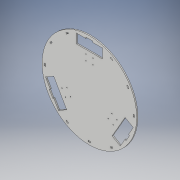
# Autodesk Inventor part: debanhxe
Saved by Autodesk Inventor 2019 (Build 230136000, 136)
## iProperties
Created: 2021-01-15
Part Number: debanhxe
Material: Generic
Document SubType Name: Modeling
Designer: Admin
Density: 1 g/cm^3
Appearance: Default
Author: Admin
Autodesk Inventor part; units mm, degrees
ref_plane "YZ Plane" through (0, 0, 0) normal (1, 0, 0) x (0, 1, 0)
ref_plane "XZ Plane" through (0, 0, 0) normal (0, 1, 0) x (-1, 0, 0)
ref_plane "XY Plane" through (0, 0, 0) normal (0, 0, 1) x (1, 0, 0)
sketch "Sketch1" plane through (0, 0, 0) normal (0, 0, 1) x (1, 0, 0)
  circle A0 centre (0, 0) radius 200
  line L0 (90.6699, 167.0448) -> (88.1699, 162.7147)
  line L1 (96.8301, 157.7147) -> (99.3301, 162.0448)
  line L2 (162.0448, 99.3301) -> (157.7147, 96.8301)
  line L3 (162.7147, 88.1699) -> (167.0448, 90.6699)
  line L4 (185, 5) -> (190, 5)
  line L5 (190, -5) -> (185, -5)
  line L6 (88.1699, -162.7147) -> (96.8301, -157.7147)
  line L7 (99.3301, -162.0448) -> (90.6699, -167.0448)
  line L8 (-5, -190) -> (-5, -185)
  line L9 (5, -185) -> (5, -190)
  line L10 (-99.3301, -162.0448) -> (-90.6699, -167.0448)
  line L11 (-88.1699, -162.7147) -> (-96.8301, -157.7147)
  line L12 (-190, 5) -> (-190, -5)
  line L13 (-190, -5) -> (-185, -5)
  line L14 (-185, -5) -> (-185, 5)
  line L15 (-167.0448, 90.6699) -> (-162.0448, 99.3301)
  line L16 (-157.7147, 96.8301) -> (-162.7147, 88.1699)
  line L17 (-99.3301, 162.0448) -> (-90.6699, 167.0448)
  line L18 (-88.1699, 162.7147) -> (-96.8301, 157.7147)
  line L19 (-190, -5) -> (-190, 5)
  line L20 (-185, 5) -> (-185, -5)
  line L21 (88.1699, 162.7147) -> (96.8301, 157.7147)
  line L22 (99.3301, 162.0448) -> (90.6699, 167.0448)
  line L23 (162.7147, 88.1699) -> (157.7147, 96.8301)
  line L24 (162.0448, 99.3301) -> (167.0448, 90.6699)
  line L25 (185, 5) -> (185, -5)
  line L26 (190, 5) -> (190, -5)
  line L27 (96.8301, -157.7147) -> (99.3301, -162.0448)
  line L28 (88.1699, -162.7147) -> (90.6699, -167.0448)
  line L29 (-5, -185) -> (5, -185)
  line L30 (-5, -190) -> (5, -190)
  line L31 (-99.3301, -162.0448) -> (-96.8301, -157.7147)
  line L32 (-90.6699, -167.0448) -> (-88.1699, -162.7147)
  line L33 (-190, 5) -> (-185, 5)
  line L34 (-162.0448, 99.3301) -> (-157.7147, 96.8301)
  line L35 (-167.0448, 90.6699) -> (-162.7147, 88.1699)
  line L36 (-99.3301, 162.0448) -> (-96.8301, 157.7147)
  line L37 (-90.6699, 167.0448) -> (-88.1699, 162.7147)
  line L38 (0, 142.5) -> (55, 142.5)
  line L39 (55, 142.5) -> (55, 182.5)
  line L40 (55, 182.5) -> (15, 182.5)
  line L41 (15, 182.5) -> (15, 187.5)
  line L42 (15, 187.5) -> (0, 187.5)
  line L43 (0, 142.5) -> (-55, 142.5)
  line L44 (-55, 142.5) -> (-55, 182.5)
  line L45 (-55, 182.5) -> (-15, 182.5)
  line L46 (-15, 182.5) -> (-15, 187.5)
  line L47 (-15, 187.5) -> (0, 187.5)
  line L48 (-123.4086, -71.25) -> (-95.9086, -118.8814)
  line L49 (-150.5496, -104.2404) -> (-154.8798, -106.7404)
  line L50 (-154.8798, -106.7404) -> (-162.3798, -93.75)
  line L51 (-95.9086, -118.8814) -> (-130.5496, -138.8814)
  line L52 (-130.5496, -138.8814) -> (-150.5496, -104.2404)
  line L53 (-123.4086, -71.25) -> (-150.9086, -23.6186)
  line L54 (-165.5496, -78.2596) -> (-169.8798, -80.7596)
  line L55 (-150.9086, -23.6186) -> (-185.5496, -43.6186)
  line L56 (-185.5496, -43.6186) -> (-165.5496, -78.2596)
  line L57 (-169.8798, -80.7596) -> (-162.3798, -93.75)
  line L58 (123.4086, -71.25) -> (150.9086, -23.6186)
  line L59 (165.5496, -78.2596) -> (169.8798, -80.7596)
  line L60 (169.8798, -80.7596) -> (162.3798, -93.75)
  line L61 (150.9086, -23.6186) -> (185.5496, -43.6186)
  line L62 (185.5496, -43.6186) -> (165.5496, -78.2596)
  line L63 (123.4086, -71.25) -> (95.9086, -118.8814)
  line L64 (150.5496, -104.2404) -> (154.8798, -106.7404)
  line L65 (95.9086, -118.8814) -> (130.5496, -138.8814)
  line L66 (130.5496, -138.8814) -> (150.5496, -104.2404)
  line L67 (154.8798, -106.7404) -> (162.3798, -93.75)
  line L68 (157.7147, 96.8301) -> (162.0448, 99.3301)
  line L69 (167.0448, 90.6699) -> (162.7147, 88.1699)
  line L70 (-99.3301, -162.0448) -> (-96.8301, -157.7147)
  line L71 (-88.1699, -162.7147) -> (-90.6699, -167.0448)
  line L72 (-99.3301, -162.0448) -> (-96.8301, -157.7147)
  line L73 (-88.1699, -162.7147) -> (-90.6699, -167.0448)
  line L74 (-99.3301, -162.0448) -> (-90.6699, -167.0448)
  circle A1 centre (14.945, 125) radius 1.73
  circle A2 centre (14.945, 100.94) radius 1.73
  circle A3 centre (-14.945, 125) radius 1.73
  circle A4 centre (-14.945, 100.94) radius 1.73
  circle A5 centre (-100.7807, -75.4427) radius 1.73
  circle A6 centre (-115.7257, -49.5573) radius 1.73
  circle A7 centre (-79.9441, -63.4127) radius 1.73
  circle A8 centre (-94.8891, -37.5273) radius 1.73
  circle A9 centre (115.7257, -49.5573) radius 1.73
  circle A10 centre (100.7807, -75.4427) radius 1.73
  circle A11 centre (94.8891, -37.5273) radius 1.73
  circle A12 centre (79.9441, -63.4127) radius 1.73
  dimension "d15" = 45
  dimension "d17" = 40
  dimension "d18" = 40
  dimension "d21" = 360
  dimension "d27" = 3.46
  dimension "d48" = 360
  constraints: 150 end point, 13 centre point, 11 equal length, 8 perpendicular, 4 vertical, 2 horizontal, 2 point on line, 86 other
  measures "d15" distance of L42.end L38.start
  measures "d17" distance of L38.end L39.end
  measures "d18" distance of L39.end L40.end
  measures "d27" diameter of A1
extrude "Extrusion1" add sketch "Sketch1" along normal blind 5 contours A0 | A1 | A2 | A3 | A4 | A5 | A6 | A7 | A8 | A9 | A10 | A11 | A12
extrude "Extrusion5" cut sketch "Sketch1" along normal blind 5 contours A1 | A2 | A3 | A4 | A5 | A6 | A7 | A8 | A9 | A10 | A11 | A12
body "Solid1"
